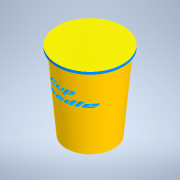
# Autodesk Inventor part: cup noodle
Saved by Autodesk Inventor 2020 (Build 240168000, 168)
## iProperties
Created: 2021-02-27
Part Number: cup noodle
Material: Generic
Document SubType Name: Modeling
Designer: Bernard Li
Density: 1 g/cm^3
Appearance: Default
Author: Bernard Li
Autodesk Inventor part; units mm, degrees
ref_plane "YZ Plane" through (0, 0, 0) normal (1, 0, 0) x (0, 1, 0)
ref_plane "XZ Plane" through (0, 0, 0) normal (0, 1, 0) x (-1, 0, 0)
ref_plane "XY Plane" through (0, 0, 0) normal (0, 0, 1) x (1, 0, 0)
sketch "Sketch1" plane through (0, 0, 0) normal (0, 0, 1) x (1, 0, 0)
  line L0 (0, 0) -> (33.5, 0)
  line L1 (0, 0) -> (33.5, 0) construction
  line L2 (0, 0) -> (0, 110)
  line L3 (0, 110) -> (46.5, 110)
  line L4 (46.5, 110) -> (46.5, 106.5)
  line L5 (46.5, 106.5) -> (43, 106.5)
  line L6 (43, 106.5) -> (33.5, 0)
  dimension "d0" = 33.5
  dimension "d1" = 0
  dimension "d2" = 110
  dimension "d3" = 46.5
  dimension "d4" = 3.5
  dimension "d5" = 3.5
  constraints: 14 end point, 3 horizontal, 3 perpendicular, 1 collinear
  measures "d0" distance of L0.start L0.end
  measures "d1" distance between parallel lines of L0 L1
  measures "d2" distance of L0.start L2.end
  measures "d3" distance of L2.end L3.end
  measures "d4" distance of L3.end L4.end
  measures "d5" distance of L4.end L5.end
revolve "Revolution1" add sketch "Sketch1" angle 360 about axis through (0, 0, 0) along (0, 1, 0)
sketch "Sketch2" plane through (0, 0, 0) normal (0, 0, 1) x (1, 0, 0)
  line L0 (-27.9354, 81.4428) -> (28.1655, 81.4428) construction
  line L1 (28.1655, 81.4428) -> (28.1655, 20.6061) construction
  line L2 (28.1655, 20.6061) -> (-27.9354, 20.6061) construction
  line L3 (-27.9354, 20.6061) -> (-27.9354, 81.4428) construction
  spline S0 degree 2 poles (-20.4896, 73.8228) (-21.4399, 73.8228) (-21.921, 75.0316) (-21.2294, 75.8676) knots 0 0 0 1 2 2 2
  line L4 (-21.2294, 75.8676) -> (-17.7231, 80.27)
  spline S1 degree 2 poles (-17.7231, 80.27) (-16.7669, 81.4308) (-15.0408, 81.4428) knots 0 0 0 1 1 1
  line L5 (-15.0408, 81.4428) -> (-8.353, 81.4428)
  spline S2 degree 2 poles (-8.353, 81.4428) (-7.517, 81.4428) (-7.072, 80.3061) (-7.4569, 79.7949) knots 0 0 0 1 2 2 2
  line L6 (-7.4569, 79.7949) -> (-8.1425, 78.8928)
  line L7 (-8.1425, 78.8928) -> (-12.3284, 78.8928)
  line L8 (-12.3284, 78.8928) -> (-12.0156, 79.2717)
  spline S3 degree 2 poles (-12.0156, 79.2717) (-11.8593, 79.4581) (-11.9615, 79.843) (-12.3584, 79.843) knots 0 0 0 1 2 2 2
  line L9 (-12.3584, 79.843) -> (-13.3087, 79.843)
  spline S4 degree 2 poles (-13.3087, 79.843) (-13.8319, 79.843) (-14.1868, 79.398) knots 0 0 0 1 1 1
  line L10 (-14.1868, 79.398) -> (-16.9713, 75.9518)
  spline S5 degree 2 poles (-16.9713, 75.9518) (-17.1097, 75.7774) (-16.9834, 75.4226) (-16.6526, 75.4226) knots 0 0 0 1 2 2 2
  line L11 (-16.6526, 75.4226) -> (-15.7204, 75.4226)
  spline S6 degree 2 poles (-15.7204, 75.4226) (-15.1129, 75.4226) (-14.7701, 75.8917) knots 0 0 0 1 1 1
  line L12 (-14.7701, 75.8917) -> (-14.3852, 76.3488)
  line L13 (-14.3852, 76.3488) -> (-10.1813, 76.3488)
  line L14 (-10.1813, 76.3488) -> (-11.2759, 74.9835)
  spline S7 degree 2 poles (-11.2759, 74.9835) (-12.184, 73.8228) (-14.0184, 73.8228) knots 0 0 0 1 1 1
  line L15 (-14.0184, 73.8228) -> (-20.4896, 73.8228)
  line L16 (0.53, 73.8228) -> (-2.435, 73.8228)
  line L17 (-2.435, 73.8228) -> (-2.2666, 74.0092)
  spline S8 degree 2 poles (-2.2666, 74.0092) (-2.7177, 73.8228) (-3.3251, 73.8228) knots 0 0 0 1 1 1
  line L18 (-3.3251, 73.8228) -> (-7.9019, 73.8228)
  spline S9 degree 2 poles (-7.9019, 73.8228) (-8.8461, 73.8228) (-9.1769, 74.9474) (-8.78, 75.5008) knots 0 0 0 1 2 2 2
  line L19 (-8.78, 75.5008) -> (-5.8691, 79.1995)
  line L20 (-5.8691, 79.1995) -> (-1.6351, 79.1995)
  line L21 (-1.6351, 79.1995) -> (-4.2814, 75.9097)
  spline S10 degree 2 poles (-4.2814, 75.9097) (-4.4919, 75.6571) (-4.3535, 75.4226) (-4.149, 75.4226) knots 0 0 0 1 2 2 2
  line L22 (-4.149, 75.4226) -> (-1.6712, 75.4226)
  spline S11 degree 2 poles (-1.6712, 75.4226) (-1.154, 75.4226) (-0.8893, 75.7654) knots 0 0 0 1 1 1
  line L23 (-0.8893, 75.7654) -> (1.8832, 79.1995)
  line L24 (1.8832, 79.1995) -> (4.7881, 79.1995)
  line L25 (4.7881, 79.1995) -> (0.53, 73.8228)
  line L26 (6.863, 79.1995) -> (11.0609, 79.1995)
  line L27 (11.0609, 79.1995) -> (10.8624, 78.977)
  spline S12 degree 2 poles (10.8624, 78.977) (11.3195, 79.1995) (12.1615, 79.1995) knots 0 0 0 1 1 1
  line L28 (12.1615, 79.1995) -> (15.337, 79.1995)
  spline S13 degree 2 poles (15.337, 79.1995) (16.185, 79.1875) (16.6, 78.0267) (16.2151, 77.5576) knots 0 0 0 1 2 2 2
  line L29 (16.2151, 77.5576) -> (14.1702, 74.9715)
  spline S14 degree 2 poles (14.1702, 74.9715) (13.238, 73.8108) (11.518, 73.8228) knots 0 0 0 1 1 1
  line L30 (11.518, 73.8228) -> (7.5065, 73.8228)
  spline S15 degree 2 poles (7.5065, 73.8228) (7.0374, 73.8228) (7.0795, 74.0754) knots 0 0 0 1 1 1
  line L31 (7.0795, 74.0754) -> (4.4392, 70.7856)
  line L32 (4.4392, 70.7856) -> (0.2052, 70.7856)
  line L33 (0.2052, 70.7856) -> (6.863, 79.1995)
  line L34 (10.682, 75.8796) -> (11.5901, 77.0284)
  spline S16 degree 2 poles (11.5901, 77.0284) (11.7345, 77.2148) (11.6322, 77.5997) (11.2533, 77.5997) knots 0 0 0 1 2 2 2
  line L35 (11.2533, 77.5997) -> (10.3392, 77.5997)
  spline S17 degree 2 poles (10.3392, 77.5997) (9.7859, 77.5817) (9.4431, 77.1547) knots 0 0 0 1 1 1
  line L36 (9.4431, 77.1547) -> (8.5109, 75.9638)
  spline S18 degree 2 poles (8.5109, 75.9638) (8.3545, 75.7654) (8.5109, 75.4286) (8.8356, 75.4226) knots 0 0 0 1 2 2 2
  line L37 (8.8356, 75.4226) -> (9.7317, 75.4226)
  spline S19 degree 2 poles (9.7317, 75.4226) (10.3572, 75.4226) (10.682, 75.8796) knots 0 0 0 1 1 1
  line L38 (-36.7039, 60.4714) -> (-30.6296, 68.0914)
  line L39 (-30.6296, 68.0914) -> (-27.4361, 68.0914)
  line L40 (-27.4361, 68.0914) -> (-26.5159, 64.2904)
  line L41 (-26.5159, 64.2904) -> (-23.4907, 68.0914)
  line L42 (-23.4907, 68.0914) -> (-20.5979, 68.0914)
  line L43 (-20.5979, 68.0914) -> (-26.6843, 60.4714)
  line L44 (-26.6843, 60.4714) -> (-30.0222, 60.4714)
  line L45 (-30.0222, 60.4714) -> (-30.9423, 64.2904)
  line L46 (-30.9423, 64.2904) -> (-33.9675, 60.4714)
  line L47 (-33.9675, 60.4714) -> (-36.7039, 60.4714)
  line L48 (-23.0036, 62.1193) -> (-20.9768, 64.6753)
  spline S20 degree 2 poles (-20.9768, 64.6753) (-20.0266, 65.8541) (-18.3486, 65.8481) knots 0 0 0 1 1 1
  line L49 (-18.3486, 65.8481) -> (-11.5766, 65.8481)
  spline S21 degree 2 poles (-11.5766, 65.8481) (-10.7286, 65.8361) (-10.3136, 64.6874) (-10.6985, 64.2183) knots 0 0 0 1 2 2 2
  line L50 (-10.6985, 64.2183) -> (-12.7433, 61.6321)
  spline S22 degree 2 poles (-12.7433, 61.6321) (-13.6695, 60.4714) (-15.4257, 60.4714) knots 0 0 0 1 1 1
  line L51 (-15.4257, 60.4714) -> (-22.1255, 60.4714)
  spline S23 degree 2 poles (-22.1255, 60.4714) (-23.0036, 60.4714) (-23.4005, 61.6201) (-23.0036, 62.1193) knots 0 0 0 1 2 2 2
  line L52 (-16.2376, 62.5283) -> (-15.3295, 63.677)
  spline S24 degree 2 poles (-15.3295, 63.677) (-15.1851, 63.8634) (-15.2874, 64.2483) (-15.6663, 64.2483) knots 0 0 0 1 2 2 2
  line L53 (-15.6663, 64.2483) -> (-16.5804, 64.2483)
  spline S25 degree 2 poles (-16.5804, 64.2483) (-17.1337, 64.2303) (-17.4825, 63.8033) knots 0 0 0 1 1 1
  line L54 (-17.4825, 63.8033) -> (-18.4087, 62.6125)
  spline S26 degree 2 poles (-18.4087, 62.6125) (-18.5651, 62.414) (-18.4087, 62.0772) (-18.084, 62.0712) knots 0 0 0 1 2 2 2
  line L55 (-18.084, 62.0712) -> (-17.1878, 62.0712)
  spline S27 degree 2 poles (-17.1878, 62.0712) (-16.5624, 62.0712) (-16.2376, 62.5283) knots 0 0 0 1 1 1
  line L56 (-10.2715, 62.1193) -> (-8.2447, 64.6753)
  spline S28 degree 2 poles (-8.2447, 64.6753) (-7.2945, 65.8541) (-5.6165, 65.8481) knots 0 0 0 1 1 1
  line L57 (-5.6165, 65.8481) -> (1.1555, 65.8481)
  spline S29 degree 2 poles (1.1555, 65.8481) (2.0035, 65.8361) (2.4185, 64.6874) (2.0336, 64.2183) knots 0 0 0 1 2 2 2
  line L58 (2.0336, 64.2183) -> (-0.0113, 61.6321)
  spline S30 degree 2 poles (-0.0113, 61.6321) (-0.9375, 60.4714) (-2.6936, 60.4714) knots 0 0 0 1 1 1
  line L59 (-2.6936, 60.4714) -> (-9.3934, 60.4714)
  spline S31 degree 2 poles (-9.3934, 60.4714) (-10.2715, 60.4714) (-10.6684, 61.6201) (-10.2715, 62.1193) knots 0 0 0 1 2 2 2
  line L60 (-3.5055, 62.5283) -> (-2.5974, 63.677)
  spline S32 degree 2 poles (-2.5974, 63.677) (-2.453, 63.8634) (-2.5553, 64.2483) (-2.9342, 64.2483) knots 0 0 0 1 2 2 2
  line L61 (-2.9342, 64.2483) -> (-3.8483, 64.2483)
  spline S33 degree 2 poles (-3.8483, 64.2483) (-4.4016, 64.2303) (-4.7505, 63.8033) knots 0 0 0 1 1 1
  line L62 (-4.7505, 63.8033) -> (-5.6767, 62.6125)
  spline S34 degree 2 poles (-5.6767, 62.6125) (-5.833, 62.414) (-5.6767, 62.0772) (-5.3519, 62.0712) knots 0 0 0 1 2 2 2
  line L63 (-5.3519, 62.0712) -> (-4.4558, 62.0712)
  spline S35 degree 2 poles (-4.4558, 62.0712) (-3.8303, 62.0712) (-3.5055, 62.5283) knots 0 0 0 1 1 1
  line L64 (2.4606, 62.1193) -> (4.4994, 64.6753)
  spline S36 degree 2 poles (4.4994, 64.6753) (5.4496, 65.8541) (7.1276, 65.8481) knots 0 0 0 1 1 1
  line L65 (7.1276, 65.8481) -> (10.9707, 65.8481)
  spline S37 degree 2 poles (10.9707, 65.8481) (11.542, 65.8481) (11.6984, 65.6196) knots 0 0 0 1 1 1
  line L66 (11.6984, 65.6196) -> (13.671, 68.0914)
  line L67 (13.671, 68.0914) -> (17.8569, 68.0914)
  line L68 (17.8569, 68.0914) -> (11.7706, 60.4714)
  line L69 (11.7706, 60.4714) -> (7.5666, 60.4714)
  line L70 (7.5666, 60.4714) -> (7.7952, 60.724)
  spline S38 degree 2 poles (7.7952, 60.724) (7.3441, 60.4714) (6.8269, 60.4714) knots 0 0 0 1 1 1
  line L71 (6.8269, 60.4714) -> (3.3386, 60.4714)
  spline S39 degree 2 poles (3.3386, 60.4714) (2.4606, 60.4714) (2.0636, 61.6201) (2.4606, 62.1193) knots 0 0 0 1 2 2 2
  line L72 (9.2265, 62.5283) -> (10.1407, 63.677)
  spline S40 degree 2 poles (10.1407, 63.677) (10.2911, 63.8634) (10.1828, 64.2483) (9.8099, 64.2483) knots 0 0 0 1 2 2 2
  line L73 (9.8099, 64.2483) -> (8.8898, 64.2483)
  spline S41 degree 2 poles (8.8898, 64.2483) (8.3364, 64.2303) (7.9936, 63.8033) knots 0 0 0 1 1 1
  line L74 (7.9936, 63.8033) -> (7.0554, 62.6125)
  spline S42 degree 2 poles (7.0554, 62.6125) (6.8991, 62.414) (7.0554, 62.0772) (7.3802, 62.0712) knots 0 0 0 1 2 2 2
  line L75 (7.3802, 62.0712) -> (8.2763, 62.0712)
  spline S43 degree 2 poles (8.2763, 62.0712) (8.9018, 62.0712) (9.2265, 62.5283) knots 0 0 0 1 1 1
  line L76 (13.8876, 60.4714) -> (19.9619, 68.0914)
  line L77 (19.9619, 68.0914) -> (24.214, 68.0914)
  line L78 (24.214, 68.0914) -> (18.1276, 60.4714)
  line L79 (18.1276, 60.4714) -> (13.8876, 60.4714)
  spline S44 degree 2 poles (22.4999, 60.4714) (21.5497, 60.4714) (21.0685, 61.6803) (21.7602, 62.5162) knots 0 0 0 1 2 2 2
  line L80 (21.7602, 62.5162) -> (23.4983, 64.6753)
  spline S45 degree 2 poles (23.4983, 64.6753) (24.4605, 65.8361) (26.1806, 65.8421) knots 0 0 0 1 1 1
  line L81 (26.1806, 65.8421) -> (32.8504, 65.8421)
  spline S46 degree 2 poles (32.8504, 65.8421) (33.6863, 65.8421) (34.1374, 64.7054) (33.7525, 64.1942) knots 0 0 0 1 2 2 2
  line L82 (33.7525, 64.1942) -> (32.6098, 62.7448)
  line L83 (32.6098, 62.7448) -> (26.1806, 62.7448)
  line L84 (26.1806, 62.7448) -> (26.0182, 62.6004)
  spline S47 degree 2 poles (26.0182, 62.6004) (25.8799, 62.42) (26.0062, 62.0652) (26.337, 62.0652) knots 0 0 0 1 2 2 2
  line L85 (26.337, 62.0652) -> (27.2692, 62.0652)
  spline S48 degree 2 poles (27.2692, 62.0652) (27.8766, 62.0652) (28.051, 62.2877) knots 0 0 0 1 1 1
  line L86 (28.051, 62.2877) -> (32.2369, 62.2877)
  line L87 (32.2369, 62.2877) -> (31.7137, 61.6261)
  spline S49 degree 2 poles (31.7137, 61.6261) (30.8055, 60.4714) (28.9712, 60.4714) knots 0 0 0 1 1 1
  line L88 (28.9712, 60.4714) -> (22.4999, 60.4714)
  spline S50 degree 2 poles (29.1576, 63.665) (29.3441, 63.8634) (29.2418, 64.2483) (28.8449, 64.2483) knots 0 0 0 1 2 2 2
  line L89 (28.8449, 64.2483) -> (27.8646, 64.2483)
  spline S51 degree 2 poles (27.8646, 64.2483) (27.3413, 64.2483) (26.9865, 63.7973) knots 0 0 0 1 1 1
  line L90 (26.9865, 63.7973) -> (26.776, 63.5387)
  line L91 (26.776, 63.5387) -> (29.0434, 63.5387)
  line L92 (29.0434, 63.5387) -> (29.1576, 63.665)
  constraints: 2 other
extrude "Extrusion1" cut sketch "Sketch2" along normal up to surface
sketch "Sketch3" plane through (0, 0, 0) normal (0, -1, 0) x (1, 0, 0)
  circle A0 centre (0, 0) radius 30.1625
  constraints: 1 centre point
extrude "Extrusion2" cut sketch "Sketch3" against normal blind 6.35
body "Solid1"
